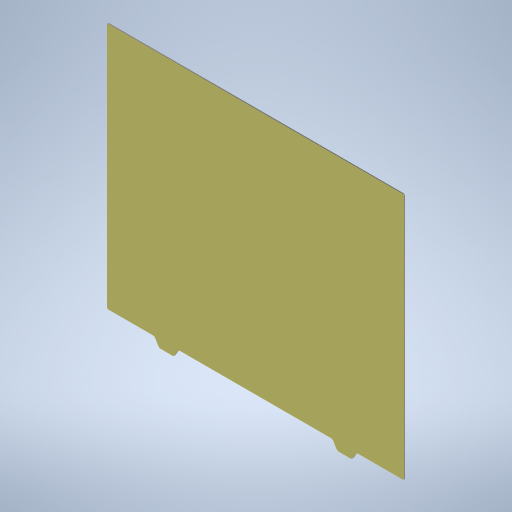
# Autodesk Inventor part: PEI Bed Surface
Saved by Autodesk Inventor 2024 (Build 280153000, 153)
## iProperties
Created: 2024-08-02
Part Number: PEI Bed Surface
Material: Steel, Alloy
Document SubType Name: Modeling
Designer: Ishaan
Density: 7.73 g/cm^3
Appearance: Semi-Polished
Author: Ishaan
Autodesk Inventor part; units mm, degrees
ref_plane "YZ Plane" through (0, 0, 0) normal (1, 0, 0) x (0, 1, 0)
ref_plane "XZ Plane" through (0, 0, 0) normal (0, 1, 0) x (-1, 0, 0)
ref_plane "XY Plane" through (0, 0, 0) normal (0, 0, 1) x (1, 0, 0)
sketch "Sketch1" plane through (0, 0, 0) normal (0, 0, 1) x (1, 0, 0)
  line L0 (150, -125) -> (-150, -125)
  line L1 (-150, -125) -> (-150, 125)
  line L2 (-150, 125) -> (150, 125)
  line L3 (150, 125) -> (150, -125)
  line L4 (150, -125) -> (-150, 125) construction
  line L5 (-150, -125) -> (150, 125) construction
  point P0 (0, 0)
  dimension "d0" = 300
  dimension "d1" = 250
  constraints: 12 end point, 2 midpoint, 2 parallel, 1 horizontal, 1 perpendicular
  measures "d0" distance of L1.end L2.end
  measures "d1" distance of L0.end L1.end
extrude "Extrusion1" add sketch "Sketch1" along normal blind 1
fillet "Fillet1" radius 1 4 edges at (-150, 125, 0.5) (-150, -125, 0.5) (150, -125, 0.5) (150, 125, 0.5)
sketch "Sketch3" plane through (0, 0, 0) normal (0, 0, -1) x (-1, 0, 0)
  line L0 (149, -125) -> (-149, -125) projected
  line L1 (102.1188, -125) -> (97.5, -133)
  line L2 (97.5, -133) -> (82.5, -133)
  line L3 (82.5, -133) -> (77.8812, -125)
  point P0 (0, 0)
  point P1 (90, -133)
  dimension "d7" = 60
  dimension "d8" = 60
  dimension "d9" = 8
  dimension "d10" = 15
  dimension "d11" = 90
  constraints: 6 end point, 2 point on line, 1 midpoint, 1 parallel
  measures "d7" angle of L0 L1
  measures "d8" angle of L0 L3
  measures "d9" distance between parallel lines of L0 L2
  measures "d10" distance of L1.end L2.end
  measures "d11" horizontal distance of point (0, 0) point (90, -133)
extrude "Extrusion3" add sketch "Sketch3" against normal up to surface (1 mm away)
mirror "Mirror1" about plane through (0, 0, 0) normal (1, 0, 0) of "Extrusion3"
fillet "Fillet2" radius 3 8 edges at (-77.8812, -125, 0.5) (-82.5, -133, 0.5) (-102.1188, -125, 0.5) (-97.5, -133, 0.5) (77.8812, -125, 0.5) (82.5, -133, 0.5) (102.1188, -125, 0.5) (97.5, -133, 0.5)
sketch "Sketch2" plane through (0, 0, 1) normal (0, 0, 1) x (1, 0, 0)
  arc A0 (150, 124) -> (149, 125) centre (149, 124) ccw projected
  line L0 (149, 125) -> (-149, 125) projected
  arc A1 (-149, 125) -> (-150, 124) centre (-149, 124) ccw projected
  line L1 (-150, 124) -> (-150, -124) projected
  arc A2 (-150, -124) -> (-149, -125) centre (-149, -124) ccw projected
  line L2 (-149, -125) -> (-103.8509, -125) projected
  arc A3 (149, -125) -> (150, -124) centre (149, -124) ccw projected
  line L3 (150, -124) -> (150, 124) projected
  arc A4 (95.7679, -133) -> (98.366, -131.5) centre (95.7679, -130) ccw projected
  line L4 (98.366, -131.5) -> (101.2528, -126.5) projected
  arc A5 (103.8509, -125) -> (101.2528, -126.5) centre (103.8509, -128) ccw projected
  line L5 (103.8509, -125) -> (149, -125) projected
  arc A6 (-101.2528, -126.5) -> (-103.8509, -125) centre (-103.8509, -128) ccw projected
  line L6 (-98.366, -131.5) -> (-101.2528, -126.5) projected
  arc A7 (-98.366, -131.5) -> (-95.7679, -133) centre (-95.7679, -130) ccw projected
  line L7 (-84.2321, -133) -> (-95.7679, -133) projected
  arc A8 (-84.2321, -133) -> (-81.634, -131.5) centre (-84.2321, -130) ccw projected
  line L8 (-78.7472, -126.5) -> (-81.634, -131.5) projected
  arc A9 (-76.1491, -125) -> (-78.7472, -126.5) centre (-76.1491, -128) ccw projected
  line L9 (-76.1491, -125) -> (76.1491, -125) projected
  arc A10 (78.7472, -126.5) -> (76.1491, -125) centre (76.1491, -128) ccw projected
  line L10 (78.7472, -126.5) -> (81.634, -131.5) projected
  arc A11 (81.634, -131.5) -> (84.2321, -133) centre (84.2321, -130) ccw projected
  line L11 (84.2321, -133) -> (95.7679, -133) projected
  point P0 (0, 0)
extrude "Extrusion2" add sketch "Sketch2" along normal blind 0.1 separate body
equation "\"d8\" = d7"
body "Solid1"
body "Solid2"
